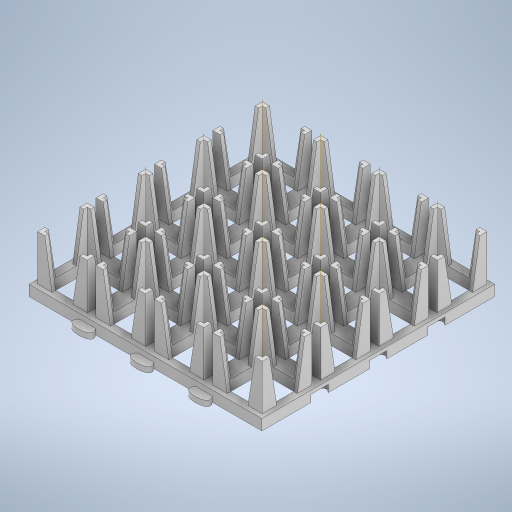
# Autodesk Inventor part: big retainer
Saved by Autodesk Inventor 2024 (Build 280153000, 153)
## iProperties
Created: 2024-03-21
Part Number: big retainer
Material: Generic
Document SubType Name: Modeling
Designer: drew
Density: 1 g/cm^3
Appearance: Default
Author: drew
Autodesk Inventor part; units mm, degrees
ref_plane "YZ Plane" through (0, 0, 0) normal (1, 0, 0) x (0, 1, 0)
ref_plane "XZ Plane" through (0, 0, 0) normal (0, 1, 0) x (-1, 0, 0)
ref_plane "XY Plane" through (0, 0, 0) normal (0, 0, 1) x (1, 0, 0)
sketch "Sketch1" plane through (0, 0, 0) normal (0, 1, 0) x (-1, 0, 0)
  line L0 (0, 0) -> (102.5144, 0)
  line L1 (102.5144, 0) -> (102.5144, -102.5144)
  line L2 (102.5144, -102.5144) -> (0, -102.5144)
  line L3 (0, -102.5144) -> (0, 0)
  line L4 (100.6602, -1.8542) -> (78.8162, -1.8542) construction
  line L5 (78.8162, -1.8542) -> (78.8162, -23.6982) construction
  line L6 (78.8162, -23.6982) -> (100.6602, -23.6982) construction
  line L7 (100.6602, -23.6982) -> (100.6602, -1.8542) construction
  line L8 (99.0727, -3.4417) -> (80.4037, -3.4417)
  line L9 (80.4037, -3.4417) -> (80.4037, -22.1107)
  line L10 (80.4037, -22.1107) -> (99.0727, -22.1107)
  line L11 (99.0727, -22.1107) -> (99.0727, -3.4417)
  line L12 (73.3552, -3.4417) -> (54.6862, -3.4417)
  line L13 (54.6862, -3.4417) -> (54.6862, -22.1107)
  line L14 (54.6862, -22.1107) -> (73.3552, -22.1107)
  line L15 (73.3552, -22.1107) -> (73.3552, -3.4417)
  line L16 (47.6377, -3.4417) -> (28.9687, -3.4417)
  line L17 (28.9687, -3.4417) -> (28.9687, -22.1107)
  line L18 (28.9687, -22.1107) -> (47.6377, -22.1107)
  line L19 (47.6377, -22.1107) -> (47.6377, -3.4417)
  line L20 (21.9202, -3.4417) -> (3.2512, -3.4417)
  line L21 (3.2512, -3.4417) -> (3.2512, -22.1107)
  line L22 (3.2512, -22.1107) -> (21.9202, -22.1107)
  line L23 (21.9202, -22.1107) -> (21.9202, -3.4417)
  line L24 (99.0727, -29.1592) -> (80.4037, -29.1592)
  line L25 (80.4037, -29.1592) -> (80.4037, -47.8282)
  line L26 (80.4037, -47.8282) -> (99.0727, -47.8282)
  line L27 (99.0727, -47.8282) -> (99.0727, -29.1592)
  line L28 (73.3552, -29.1592) -> (54.6862, -29.1592)
  line L29 (54.6862, -29.1592) -> (54.6862, -47.8282)
  line L30 (54.6862, -47.8282) -> (73.3552, -47.8282)
  line L31 (73.3552, -47.8282) -> (73.3552, -29.1592)
  line L32 (47.6377, -29.1592) -> (28.9687, -29.1592)
  line L33 (28.9687, -29.1592) -> (28.9687, -47.8282)
  line L34 (28.9687, -47.8282) -> (47.6377, -47.8282)
  line L35 (47.6377, -47.8282) -> (47.6377, -29.1592)
  line L36 (21.9202, -29.1592) -> (3.2512, -29.1592)
  line L37 (3.2512, -29.1592) -> (3.2512, -47.8282)
  line L38 (3.2512, -47.8282) -> (21.9202, -47.8282)
  line L39 (21.9202, -47.8282) -> (21.9202, -29.1592)
  line L40 (99.0727, -54.8767) -> (80.4037, -54.8767)
  line L41 (80.4037, -54.8767) -> (80.4037, -73.5457)
  line L42 (80.4037, -73.5457) -> (99.0727, -73.5457)
  line L43 (99.0727, -73.5457) -> (99.0727, -54.8767)
  line L44 (73.3552, -54.8767) -> (54.6862, -54.8767)
  line L45 (54.6862, -54.8767) -> (54.6862, -73.5457)
  line L46 (54.6862, -73.5457) -> (73.3552, -73.5457)
  line L47 (73.3552, -73.5457) -> (73.3552, -54.8767)
  line L48 (47.6377, -54.8767) -> (28.9687, -54.8767)
  line L49 (28.9687, -54.8767) -> (28.9687, -73.5457)
  line L50 (28.9687, -73.5457) -> (47.6377, -73.5457)
  line L51 (47.6377, -73.5457) -> (47.6377, -54.8767)
  line L52 (21.9202, -54.8767) -> (3.2512, -54.8767)
  line L53 (3.2512, -54.8767) -> (3.2512, -73.5457)
  line L54 (3.2512, -73.5457) -> (21.9202, -73.5457)
  line L55 (21.9202, -73.5457) -> (21.9202, -54.8767)
  line L56 (99.0727, -80.5942) -> (80.4037, -80.5942)
  line L57 (80.4037, -80.5942) -> (80.4037, -99.2632)
  line L58 (80.4037, -99.2632) -> (99.0727, -99.2632)
  line L59 (99.0727, -99.2632) -> (99.0727, -80.5942)
  line L60 (73.3552, -80.5942) -> (54.6862, -80.5942)
  line L61 (54.6862, -80.5942) -> (54.6862, -99.2632)
  line L62 (54.6862, -99.2632) -> (73.3552, -99.2632)
  line L63 (73.3552, -99.2632) -> (73.3552, -80.5942)
  line L64 (47.6377, -80.5942) -> (28.9687, -80.5942)
  line L65 (28.9687, -80.5942) -> (28.9687, -99.2632)
  line L66 (28.9687, -99.2632) -> (47.6377, -99.2632)
  line L67 (47.6377, -99.2632) -> (47.6377, -80.5942)
  line L68 (21.9202, -80.5942) -> (3.2512, -80.5942)
  line L69 (3.2512, -80.5942) -> (3.2512, -99.2632)
  line L70 (3.2512, -99.2632) -> (21.9202, -99.2632)
  line L71 (21.9202, -99.2632) -> (21.9202, -80.5942)
  dimension "d0" = 102.5144
  dimension "d1" = 21.844
  dimension "d2" = 1.8542
  dimension "d3" = 1.8542
  dimension "d4" = 1.5875
  dimension "d7" = 25.7175
  dimension "d10" = 25.7175
  constraints: 144 end point, 6 parallel, 5 perpendicular, 3 horizontal, 1 vertical, 123 other
  measures "d0" distance of L0.end L1.end
  measures "d1" distance of L6.end L4.start
  measures "d2" distance between parallel lines of L1 L7
  measures "d3" distance between parallel lines of L0 L4
  measures "d4" distance between parallel lines of L7 L11
  measures "d7" distance of L8.start L12.start
  measures "d10" distance of L8.start L24.start
extrude "Extrusion1" add sketch "Sketch1" along normal blind 4.7625
sketch "Sketch2" plane through (0, 4.7625, 0) normal (0, 1, 0) x (1, 0, 0)
  line L0 (-99.0727, 3.4417) -> (-99.0727, 22.1107) projected
  line L1 (-80.4037, 3.4417) -> (-99.0727, 3.4417) projected
  line L2 (-80.4037, 22.1107) -> (-80.4037, 3.4417) projected
  line L3 (-99.0727, 22.1107) -> (-80.4037, 22.1107) projected
  line L4 (-100.6602, 23.6982) -> (-100.6602, 1.8542)
  line L5 (-100.6602, 1.8542) -> (-78.8162, 1.8542)
  line L6 (-78.8162, 1.8542) -> (-78.8162, 23.6982)
  line L7 (-78.8162, 23.6982) -> (-100.6602, 23.6982)
  point P0 (0, 0)
  dimension "d15" = 21.844
  constraints: 8 end point, 3 other
  measures "d15" distance of L4.start L4.end
extrude "Extrusion2" add sketch "Sketch2" along normal blind 20.066
sketch "Sketch3" plane through (-100.6602, 4.7625, -1.8542) normal (0, 0, 1) x (1, 0, 0)
  line L0 (21.844, 0) -> (0, 0) projected
  line L1 (21.844, 0) -> (21.844, 20.066) projected
  line L2 (0, 20.066) -> (21.844, 20.066) projected
  line L3 (0, 0) -> (0, 20.066) projected
  line L4 (-1.8542, 0) -> (100.6602, 0) projected
  line L5 (6.35, 0) -> (3.175, 20.066)
  line L6 (15.494, 0) -> (18.669, 20.066)
  point P0 (100.6602, -4.7625)
  point P1 (15.494, 0)
  point P2 (6.35, 0)
  dimension "d18" = 6.35
  dimension "d19" = 6.35
  dimension "d20" = 3.175
  dimension "d21" = 3.175
  constraints: 4 end point, 4 point on line
  measures "d18" distance from line of L3 L5.start
  measures "d19" distance from line of L1 L6.start
  measures "d20" distance from line of L1 L6.end
  measures "d21" distance from line of L3 L5.end
extrude "Extrusion3" cut sketch "Sketch3" against normal up to surface (21.844 mm away) contours L0 L5 L2 L6
sketch "Sketch4" plane through (0, 24.8285, 0) normal (0, 1, 0) x (1, 0, 0)
  line L0 (-97.4852, 22.1107) -> (-97.4852, 23.6982) projected
  line L1 (-97.4852, 23.6982) -> (-100.6602, 23.6982) projected
  line L2 (-100.6602, 23.6982) -> (-100.6602, 1.8542) projected
  line L3 (-100.6602, 1.8542) -> (-97.4852, 1.8542) projected
  line L4 (-97.4852, 1.8542) -> (-97.4852, 3.4417) projected
  line L5 (-97.4852, 3.4417) -> (-99.0727, 3.4417) projected
  line L6 (-99.0727, 3.4417) -> (-99.0727, 22.1107) projected
  line L7 (-99.0727, 22.1107) -> (-97.4852, 22.1107) projected
  line L8 (-81.9912, 23.6982) -> (-81.9912, 22.1107) projected
  line L9 (-81.9912, 22.1107) -> (-80.4037, 22.1107) projected
  line L10 (-80.4037, 22.1107) -> (-80.4037, 3.4417) projected
  line L11 (-80.4037, 3.4417) -> (-81.9912, 3.4417) projected
  line L12 (-81.9912, 3.4417) -> (-81.9912, 1.8542) projected
  line L13 (-81.9912, 1.8542) -> (-78.8162, 1.8542) projected
  line L14 (-78.8162, 1.8542) -> (-78.8162, 23.6982) projected
  line L15 (-78.8162, 23.6982) -> (-81.9912, 23.6982) projected
  line L16 (-80.4037, 3.4417) -> (-99.0727, 22.1107) construction
  line L17 (-99.0727, 3.4417) -> (-80.4037, 22.1107) construction
  point P0 (0, 0)
  point P1 (-89.7382, 12.7762)
  constraints: 4 end point, 1 midpoint
pattern_circular "Circular Pattern1" count 2 over 90 about axis through (-89.7382, 24.8285, -12.7762) along (0, 1, 0) of "Extrusion3"
pattern_linear "Rectangular Pattern1" count 4 spacing 25.7175 along (0, 0, -1) count 4 spacing 25.7175 along (1, 0, 0) of "Extrusion2", "Extrusion3", "Circular Pattern1"
sketch "Sketch5" plane through (0, 0, 0) normal (0, -1, 0) x (1, 0, 0)
  line L0 (0, -102.5144) -> (-102.5144, -102.5144) projected
  line L1 (0, 0) -> (0, -102.5144) projected
  line L2 (-102.5144, 0) -> (0, 0) projected
  line L3 (-102.5144, -102.5144) -> (-102.5144, 0) projected
  line L4 (-21.9202, -80.5942) -> (-21.9202, -99.2632) projected
  line L5 (-3.2512, -80.5942) -> (-21.9202, -80.5942) projected
  line L6 (-3.2512, -99.2632) -> (-3.2512, -80.5942) projected
  line L7 (-21.9202, -99.2632) -> (-3.2512, -99.2632) projected
  line L8 (-47.6377, -80.5942) -> (-47.6377, -99.2632) projected
  line L9 (-28.9687, -80.5942) -> (-47.6377, -80.5942) projected
  line L10 (-28.9687, -99.2632) -> (-28.9687, -80.5942) projected
  line L11 (-47.6377, -99.2632) -> (-28.9687, -99.2632) projected
  line L12 (-73.3552, -80.5942) -> (-73.3552, -99.2632) projected
  line L13 (-54.6862, -80.5942) -> (-73.3552, -80.5942) projected
  line L14 (-54.6862, -99.2632) -> (-54.6862, -80.5942) projected
  line L15 (-73.3552, -99.2632) -> (-54.6862, -99.2632) projected
  line L16 (-99.0727, -80.5942) -> (-99.0727, -99.2632) projected
  line L17 (-80.4037, -80.5942) -> (-99.0727, -80.5942) projected
  line L18 (-80.4037, -99.2632) -> (-80.4037, -80.5942) projected
  line L19 (-99.0727, -99.2632) -> (-80.4037, -99.2632) projected
  line L20 (-21.9202, -54.8767) -> (-21.9202, -73.5457) projected
  line L21 (-3.2512, -54.8767) -> (-21.9202, -54.8767) projected
  line L22 (-3.2512, -73.5457) -> (-3.2512, -54.8767) projected
  line L23 (-21.9202, -73.5457) -> (-3.2512, -73.5457) projected
  line L24 (-47.6377, -54.8767) -> (-47.6377, -73.5457) projected
  line L25 (-28.9687, -54.8767) -> (-47.6377, -54.8767) projected
  line L26 (-28.9687, -73.5457) -> (-28.9687, -54.8767) projected
  line L27 (-47.6377, -73.5457) -> (-28.9687, -73.5457) projected
  line L28 (-73.3552, -54.8767) -> (-73.3552, -73.5457) projected
  line L29 (-54.6862, -54.8767) -> (-73.3552, -54.8767) projected
  line L30 (-54.6862, -73.5457) -> (-54.6862, -54.8767) projected
  line L31 (-73.3552, -73.5457) -> (-54.6862, -73.5457) projected
  line L32 (-99.0727, -54.8767) -> (-99.0727, -73.5457) projected
  line L33 (-80.4037, -54.8767) -> (-99.0727, -54.8767) projected
  line L34 (-80.4037, -73.5457) -> (-80.4037, -54.8767) projected
  line L35 (-99.0727, -73.5457) -> (-80.4037, -73.5457) projected
  line L36 (-21.9202, -29.1592) -> (-21.9202, -47.8282) projected
  line L37 (-3.2512, -29.1592) -> (-21.9202, -29.1592) projected
  line L38 (-3.2512, -47.8282) -> (-3.2512, -29.1592) projected
  line L39 (-21.9202, -47.8282) -> (-3.2512, -47.8282) projected
  line L40 (-47.6377, -29.1592) -> (-47.6377, -47.8282) projected
  line L41 (-28.9687, -29.1592) -> (-47.6377, -29.1592) projected
  line L42 (-28.9687, -47.8282) -> (-28.9687, -29.1592) projected
  line L43 (-47.6377, -47.8282) -> (-28.9687, -47.8282) projected
  line L44 (-73.3552, -29.1592) -> (-73.3552, -47.8282) projected
  line L45 (-54.6862, -29.1592) -> (-73.3552, -29.1592) projected
  line L46 (-54.6862, -47.8282) -> (-54.6862, -29.1592) projected
  line L47 (-73.3552, -47.8282) -> (-54.6862, -47.8282) projected
  line L48 (-99.0727, -29.1592) -> (-99.0727, -47.8282) projected
  line L49 (-80.4037, -29.1592) -> (-99.0727, -29.1592) projected
  line L50 (-80.4037, -47.8282) -> (-80.4037, -29.1592) projected
  line L51 (-99.0727, -47.8282) -> (-80.4037, -47.8282) projected
  line L52 (-21.9202, -3.4417) -> (-21.9202, -22.1107) projected
  line L53 (-3.2512, -3.4417) -> (-21.9202, -3.4417) projected
  line L54 (-3.2512, -22.1107) -> (-3.2512, -3.4417) projected
  line L55 (-21.9202, -22.1107) -> (-3.2512, -22.1107) projected
  line L56 (-47.6377, -3.4417) -> (-47.6377, -22.1107) projected
  line L57 (-28.9687, -3.4417) -> (-47.6377, -3.4417) projected
  line L58 (-28.9687, -22.1107) -> (-28.9687, -3.4417) projected
  line L59 (-47.6377, -22.1107) -> (-28.9687, -22.1107) projected
  line L60 (-73.3552, -3.4417) -> (-73.3552, -22.1107) projected
  line L61 (-54.6862, -3.4417) -> (-73.3552, -3.4417) projected
  line L62 (-54.6862, -22.1107) -> (-54.6862, -3.4417) projected
  line L63 (-73.3552, -22.1107) -> (-54.6862, -22.1107) projected
  line L64 (-99.0727, -3.4417) -> (-99.0727, -22.1107) projected
  line L65 (-80.4037, -3.4417) -> (-99.0727, -3.4417) projected
  line L66 (-80.4037, -22.1107) -> (-80.4037, -3.4417) projected
  line L67 (-99.0727, -22.1107) -> (-80.4037, -22.1107) projected
  spline S0 degree 3 poles (-80.4037, 0) (-85.7676, 5.1769) (-67.9913, 5.1769) (-73.3552, 0) knots 0 0 0 0 1 1 1 1
  line L68 (-80.4037, -22.1107) -> (-80.4037, -3.4417) projected
  line L69 (-73.3552, -3.4417) -> (-73.3552, -22.1107) projected
  spline S1 degree 3 poles (-54.6862, 0) (-60.0501, 5.1769) (-42.2738, 5.1769) (-47.6377, 0) knots 0 0 0 0 1 1 1 1
  spline S2 degree 3 poles (-28.9687, 0) (-34.3326, 5.1769) (-16.5563, 5.1769) (-21.9202, 0) knots 0 0 0 0 1 1 1 1
  point P0 (-80.4037, 3.175)
  point P1 (-73.3552, 3.175)
  point P2 (-54.6862, 3.175)
  point P3 (-47.6377, 3.175)
  point P4 (-28.9687, 3.175)
  point P5 (-21.9202, 3.175)
  point P6 (-21.9202, 0)
  point P7 (-28.9687, 0)
  point P8 (-47.6377, 0)
  point P9 (-54.6862, 0)
  dimension "d33" = 3.175
  dimension "d36" = 25.7175
  constraints: 6 point on line, 3 horizontal, 1 horizontal alignment, 20 other
  measures "d33" distance from line of L2 point (-73.355, 3.175)
  measures "d36" distance of point (-80.404, 0) point (-54.686, 0)
extrude "Extrusion4" add sketch "Sketch5" against normal blind 2.3813 contours L2 S2 | S0 L2 | L2 S1
sketch "Sketch6" plane through (0, 0, 0) normal (0, -1, 0) x (1, 0, 0)
  spline S0 degree 3 poles (0, -21.9202) (-5.1769, -16.5563) (-5.1769, -34.3326) (0, -28.9687) knots 0 0 0 0 1 1 1 1
  spline S1 degree 3 poles (0, -47.6377) (-5.1769, -42.2738) (-5.1769, -60.0501) (0, -54.6862) knots 0 0 0 0 1 1 1 1
  spline S2 degree 3 poles (0, -73.3552) (-5.1769, -67.9913) (-5.1769, -85.7676) (0, -80.4037) knots 0 0 0 0 1 1 1 1
  line L0 (0, -80.4037) -> (0, -21.9202)
  line L1 (0, 0) -> (0, -102.5144) projected
  spline S3 degree 5 poles (0.1439, -21.7813) (-0.1302, -21.4961) (-0.4269, -21.2339) (-0.7429, -20.9939) (-1.3717, -20.6704) (-2.071, -20.6761) (-2.3614, -20.7667) (-2.8854, -21.0989) (-3.2506, -21.6019) (-3.4042, -21.8878) (-3.6891, -22.5442) (-3.8668, -23.2384) (-3.9421, -23.6224) (-4.0558, -24.4252) (-4.0922, -25.2347) (-4.0923, -25.6542) (-4.0558, -26.4637) (-3.9421, -27.2665) (-3.8668, -27.6505) (-3.6891, -28.3447) (-3.4042, -29.0011) (-3.2506, -29.287) (-2.8854, -29.79) (-2.3614, -30.1222) (-2.071, -30.2128) (-1.3717, -30.2185) (-0.7429, -29.895) (-0.4269, -29.655) (-0.1302, -29.3928) (0.1439, -29.1076) knots 0 0 0 0 0 0 0.123104 0.123104 0.123104 0.212502 0.212502 0.212502 0.313068 0.313068 0.313068 0.4348 0.4348 0.4348 0.565199 0.565199 0.565199 0.686932 0.686932 0.686932 0.787497 0.787497 0.787497 0.876896 0.876896 0.876896 1 1 1 1 1 1
  spline S4 degree 5 poles (0.1439, -47.4988) (-0.1302, -47.2136) (-0.4269, -46.9514) (-0.7429, -46.7114) (-1.3717, -46.3879) (-2.071, -46.3936) (-2.3614, -46.4842) (-2.8854, -46.8164) (-3.2506, -47.3194) (-3.4042, -47.6053) (-3.6891, -48.2617) (-3.8668, -48.9559) (-3.9421, -49.3399) (-4.0558, -50.1427) (-4.0922, -50.9522) (-4.0922, -51.3717) (-4.0558, -52.1812) (-3.9421, -52.984) (-3.8668, -53.368) (-3.6891, -54.0622) (-3.4042, -54.7186) (-3.2506, -55.0045) (-2.8854, -55.5075) (-2.3614, -55.8397) (-2.071, -55.9303) (-1.3717, -55.936) (-0.7429, -55.6125) (-0.4269, -55.3725) (-0.1302, -55.1103) (0.1439, -54.8251) knots 0 0 0 0 0 0 0.123104 0.123104 0.123104 0.212503 0.212503 0.212503 0.313068 0.313068 0.313068 0.4348 0.4348 0.4348 0.5652 0.5652 0.5652 0.686932 0.686932 0.686932 0.787497 0.787497 0.787497 0.876896 0.876896 0.876896 1 1 1 1 1 1
  spline S5 degree 5 poles (0.1439, -73.2163) (-0.1302, -72.9311) (-0.4269, -72.6689) (-0.7429, -72.4289) (-1.3717, -72.1054) (-2.071, -72.1111) (-2.3614, -72.2017) (-2.8854, -72.5339) (-3.2506, -73.0369) (-3.4042, -73.3228) (-3.6891, -73.9792) (-3.8668, -74.6734) (-3.9421, -75.0574) (-4.0558, -75.8602) (-4.0922, -76.6697) (-4.0922, -77.0892) (-4.0558, -77.8987) (-3.9421, -78.7015) (-3.8668, -79.0855) (-3.6891, -79.7797) (-3.4042, -80.4361) (-3.2506, -80.722) (-2.8854, -81.225) (-2.3614, -81.5572) (-2.071, -81.6478) (-1.3717, -81.6535) (-0.7429, -81.33) (-0.4269, -81.09) (-0.1302, -80.8278) (0.1439, -80.5426) knots 0 0 0 0 0 0 0.123104 0.123104 0.123104 0.212503 0.212503 0.212503 0.313068 0.313068 0.313068 0.4348 0.4348 0.4348 0.5652 0.5652 0.5652 0.686932 0.686932 0.686932 0.787497 0.787497 0.787497 0.876896 0.876896 0.876896 1 1 1 1 1 1
  point P0 (0, -28.9687)
  point P1 (0, -54.6862)
  point P2 (0, -80.6872)
  point P3 (0, -73.0717)
  point P4 (0, -47.3542)
  point P5 (0, -54.9697)
  point P6 (0, -21.6367)
  point P7 (0, -29.2522)
  dimension "d43" = 0.2
  dimension "d44" = 0.2
  dimension "d45" = 0.2
  dimension "d48" = 90
  constraints: 6 horizontal alignment, 2 end point, 1 collinear, 34 other
extrude "Extrusion5" cut sketch "Sketch6" against normal blind 3.175
body "Solid1"
